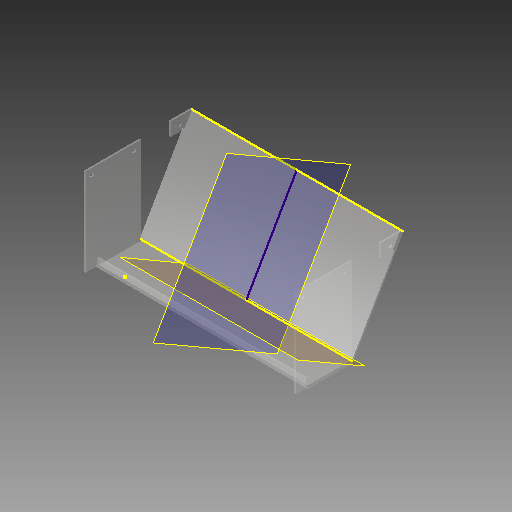
# Autodesk Inventor part: 15102898-16-P-0203
Saved by Autodesk Inventor 2017 (Build 210142000, 142)
## iProperties
Created: 2016-10-01
Part Number: 15102898-16-P-0203
Material: Polycarbonate, Clear
Document SubType Name: Modeling
Designer: Sofia
Density: 1.2 g/cm^3
Appearance: Polycarbonate - Clear
Mass: 577.727 g
Surface Area: 3131.73 cm^2
Volume: 481.439 cm^3
Author: Sofia
Autodesk Inventor part; units mm, degrees
ref_plane "YZ Plane" through (0, 0, 0) normal (1, 0, 0) x (0, 1, 0)
ref_plane "XZ Plane" through (0, 0, 0) normal (0, 1, 0) x (-1, 0, 0)
ref_plane "XY Plane" through (0, 0, 0) normal (0, 0, 1) x (1, 0, 0)
sketch "Sketch1" plane through (0, 0, 0) normal (0, 1, 0) x (-1, 0, 0)
  line L0 (0, 0) -> (-400.05, 0)
  line L1 (-400.05, 0) -> (-400.05, -107.95)
  line L2 (-400.05, -107.95) -> (0, -107.95)
  line L3 (0, -107.95) -> (0, 0)
  dimension "d0" = 400.05
  dimension "d40" = 107.95
  constraints: 8 end point, 2 parallel, 1 horizontal, 1 perpendicular
  measures "d0" distance of L2.end L1.end
  measures "d40" distance of L2.end L0.start
extrude "Extrusion1" add sketch "Sketch1" along normal blind 3.175
sketch "Sketch2" plane through (0, 3.175, 0) normal (0, 1, 0) x (1, 0, 0)
  line L0 (0, 0) -> (400.05, 0) projected
  line L1 (3.175, 0) -> (3.175, 104.775)
  line L2 (3.175, 104.775) -> (396.875, 104.775)
  line L3 (396.875, 104.775) -> (396.875, 0)
  line L4 (400.05, 0) -> (400.05, 107.95) projected
  line L5 (0, 107.95) -> (0, 0) projected
  line L6 (400.05, 107.95) -> (0, 107.95) projected
  line L7 (0, 0) -> (3.175, 0)
  line L8 (400.05, 0) -> (396.875, 0)
  line L9 (3.175, 104.775) -> (0, 104.775)
  line L10 (396.875, 104.775) -> (400.05, 104.775)
  dimension "d3" = 3.175
  dimension "d4" = 3.175
  dimension "d5" = 3.175
  constraints: 14 end point, 4 point on line, 3 perpendicular, 2 collinear, 1 vertical
  measures "d3" distance between parallel lines of L4 L3
  measures "d4" distance between parallel lines of L1 L5
  measures "d5" distance between parallel lines of L6 L2
extrude "Extrusion6" add sketch "Sketch2" along normal blind 165.1 contours L5 L9 L1 L0 | L3 L10 L4 L0
ref_plane "Work Plane1" through (400.05, 3.175, -107.95) normal (0, 0.866, -0.5) x (-1, 0, 0)
sketch "Sketch9" plane through (400.05, 3.175, -107.95) normal (0, 0.866, -0.5) x (-1, 0, 0)
  line L0 (0, 91.8999) -> (0, -1.5875) projected
  line L1 (400.05, 0) -> (0, 0)
  line L2 (0, 0) -> (0, 3.175)
  line L3 (0, 3.175) -> (400.05, 3.175)
  line L4 (400.05, 3.175) -> (400.05, 0)
  point P0 (400.05, 91.8999)
  dimension "d25" = 3.175
  constraints: 8 end point, 2 parallel, 1 coincident, 1 horizontal, 1 perpendicular, 1 point on line
  measures "d25" distance between parallel lines of L3 L1
extrude "Extrusion7" add sketch "Sketch9" along normal blind 190.6524
sketch "Sketch12" plane through (400.05, 3.175, -107.95) normal (1, 0, 0) x (0, -0.5, -0.866)
  line L0 (-3.175, 190.6524) -> (-37.872, 170.6201)
  line L1 (-37.872, 170.6201) -> (-25.172, 148.623)
  line L2 (-25.172, 148.623) -> (-3.175, 161.323)
  line L3 (-3.175, 0) -> (-3.175, 190.6524) projected
  point P0 (-91.8999, -56.7246)
  dimension "d34" = 25.4
  dimension "d35" = 60
  dimension "d36" = 25.4
  constraints: 6 end point, 1 parallel, 1 perpendicular, 1 point on line
  measures "d34" distance of L0.end L1.end
  measures "d35" angle of L3 L0
  measures "d36" distance of L1.end L2.end
extrude "Extrusion9" add sketch "Sketch12" against normal blind 3.175
sketch "Sketch13" plane through (0, 4.7625, -105.2004) normal (0, 0.5, 0.866) x (1, 0, 0)
  line L0 (400.05, 190.6524) -> (0, 190.6524) projected
  line L1 (200.025, 190.6524) -> (200.025, 0)
  line L2 (400.05, 0) -> (0, 0) projected
  point P0 (0, -56.7246)
  constraints: 2 end point, 2 midpoint
ref_plane "Work Plane2" through (200.025, 169.8723, -200.5266) normal (-1, 0, 0) x (0, -0.866, 0.5)
mirror "Mirror1" about plane through (200.025, 169.8723, -200.5266) normal (-1, 0, 0) of "Extrusion9"
sketch "Sketch14" plane through (0, 144.4723, -160.4619) normal (-1, 0, 0) x (0, 0, 1)
  circle A0 centre (-17.3381, 11.1252) radius 3.175
  line L0 (0, 0) -> (0, 25.4) projected
  line L1 (0, 25.4) -> (-40.0647, 25.4) projected
  point P0 (160.4619, -144.4723)
  dimension "d41" = 6.35
  dimension "d42" = 17.3381
  dimension "d43" = 14.2748
  constraints: 1 centre point
  measures "d41" diameter of A0
  measures "d42" distance from line of L0 A0.centre
  measures "d43" distance from line of L1 A0.centre
extrude "Extrusion10" cut sketch "Sketch14" against normal blind 431.8
sketch "Sketch16" plane through (0, 3.175, 0) normal (0, 1, 0) x (1, 0, 0)
  line L0 (400.05, 0) -> (400.05, 104.775) projected
  line L1 (0, 0) -> (400.05, 0)
  line L2 (400.05, 0) -> (400.05, 22.225)
  line L3 (400.05, 22.225) -> (0, 22.225)
  line L4 (0, 22.225) -> (0, 0)
  dimension "d49" = 22.225
  constraints: 8 end point, 2 parallel, 1 horizontal, 1 perpendicular, 1 point on line
  measures "d49" distance between parallel lines of L1 L3
extrude "Extrusion12" cut sketch "Sketch16" against normal blind 3.175
sketch "Sketch17" plane through (0, 3.175, 0) normal (0, 1, 0) x (1, 0, 0)
  line L0 (3.175, 0) -> (3.175, 104.775) projected
  line L1 (400.05, 22.225) -> (400.05, 107.95) projected
  line L2 (3.175, 22.225) -> (400.05, 22.225)
  line L3 (400.05, 22.225) -> (400.05, 25.4)
  line L4 (400.05, 25.4) -> (3.175, 25.4)
  line L5 (3.175, 25.4) -> (3.175, 22.225)
  line L6 (3.175, 22.225) -> (396.875, 22.225) projected
  point P0 (0, 0)
  dimension "d52" = 3.175
  constraints: 8 end point, 2 parallel, 2 point on line, 1 collinear, 1 horizontal, 1 perpendicular
  measures "d52" distance between parallel lines of L2 L4
extrude "Extrusion13" add sketch "Sketch17" along normal blind 12.7
sketch "Sketch18" plane through (0, 3.175, -104.775) normal (-1, 0, 0) x (0, 0, 1)
  circle A0 centre (12.7, 152.4) radius 3.175
  circle A1 centre (92.075, 152.4) radius 3.175
  line L0 (104.775, 0) -> (104.775, 165.1) projected
  line L1 (0, 0) -> (0, 165.1) projected
  line L2 (104.775, 165.1) -> (0, 165.1) projected
  point P0 (104.775, -3.175)
  dimension "d55" = 6.35
  dimension "d56" = 6.35
  dimension "d57" = 12.7
  dimension "d58" = 12.7
  dimension "d59" = 12.7
  dimension "d60" = 12.7
  constraints: 2 centre point
  measures "d55" diameter of A1
  measures "d56" diameter of A0
  measures "d57" distance from line of L0 A1.centre
  measures "d58" distance from line of L1 A0.centre
  measures "d59" distance from line of L2 A1.centre
  measures "d60" distance from line of L2 A0.centre
extrude "Extrusion14" cut sketch "Sketch18" against normal blind 508
body "Solid1"
